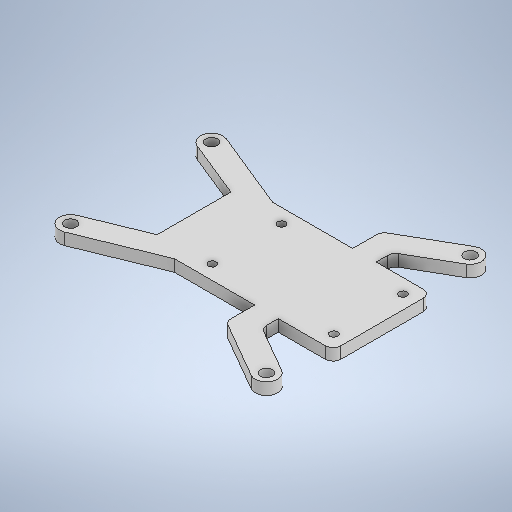
# Autodesk Inventor part: base_c
Saved by Autodesk Inventor 2025.2 (Build 292293000, 293)
## iProperties
Created: 2025-03-26
Part Number: base_c
Material: Generic
Document SubType Name: Modeling
Designer: cdavi
Density: 1 g/cm^3
Appearance: Default
Mass: 4.94389 g
Surface Area: 44.1455 cm^2
Volume: 4.94389 cm^3
Author: cdavi
Autodesk Inventor part; units mm, degrees
ref_plane "YZ Plane" through (0, 0, 0) normal (1, 0, 0) x (0, 1, 0)
ref_plane "XZ Plane" through (0, 0, 0) normal (0, 1, 0) x (-1, 0, 0)
ref_plane "XY Plane" through (0, 0, 0) normal (0, 0, 1) x (1, 0, 0)
sketch "Sketch1" plane through (0, 0, 0) normal (0, 1, 0) x (-1, 0, 0)
  line L0 (-29, 26) -> (29, 26)
  line L1 (29, 26) -> (29, -26)
  line L2 (29, -26) -> (-29, -26)
  line L3 (-29, -26) -> (-29, 26)
  line L4 (-29, 26) -> (29, -26) construction
  line L5 (29, 26) -> (-29, -26) construction
  line L6 (-32.5, 29.5) -> (32.5, 29.5)
  line L7 (32.5, -29.5) -> (-32.5, -29.5)
  line L8 (-32.5, -29.5) -> (-32.5, 29.5)
  line L9 (-32.5, 29.5) -> (32.5, -29.5) construction
  line L10 (32.5, 29.5) -> (-32.5, -29.5) construction
  circle A0 centre (-29, 26) radius 1.5
  circle A1 centre (-29, -26) radius 1.5
  line L11 (32.5, 29.5) -> (32.5, 5.9791)
  line L12 (32.5, -5.9791) -> (32.5, -29.5)
  line L13 (29, 0) -> (29, -18)
  circle A2 centre (29, -18) radius 1.5
  arc A3 (32.5, 5.9791) -> (32.5, -5.9791) centre (33, 0) ccw
  line L14 (32.5, -5.9791) -> (32.5, 5.9791)
  line L15 (33, 0) -> (-32.5, 0)
  line L16 (29, 0) -> (29, 18)
  circle A4 centre (29, 18) radius 1.5
  point P0 (0, 0)
  dimension "d1" = 58
  dimension "d3" = 3.5
  dimension "d7" = 3
  dimension "d8" = 3
  dimension "d31" = 52
  dimension "d32" = 3.5
  dimension "d33" = 18
  dimension "d34" = 3
  constraints: 34 end point, 6 midpoint, 5 centre point, 5 parallel, 4 coincident, 3 perpendicular, 2 horizontal, 2 point on circle, 2 symmetric about line, 1 point on line, 1 vertical, 2 other
  measures "d1" distance of L0.start L0.end
  measures "d3" distance between parallel lines of L7 L2
  measures "d7" diameter of A0
  measures "d8" diameter of A1
  measures "d31" distance of L0.end L1.end
  measures "d32" distance between parallel lines of L1 L11
  measures "d33" distance of L13.start L13.end
  measures "d34" diameter of A2
ref_plane "Work Plane1" through (0, 3, 0) normal (0, 1, 0) x (1, 0, 0)
extrude "Extrusion4" add sketch "Sketch1" along normal blind 3 contours A0 L3 L15 L8 L6 L11 A3 L1 A4 L0 | L0 L1 A4 A3 L15 L3 A0 | L15 A3 L1 A2 L2 A1 L3 | L3 A1 L2 L1 A2 A3 L12 L7 L8 L15
sketch "Sketch3" plane through (0, 3, 0) normal (0, 1, 0) x (1, 0, 0)
  circle A0 centre (-29, 18) radius 1.5 projected
  circle A1 centre (-29, 18) radius 2.85
  circle A2 centre (29, 26) radius 1.5 projected
  line L0 (32.5, -29.5) -> (32.5, 29.5) projected
  line L1 (32.5, 0) -> (-15.5, 0)
  line L2 (-15.5, 0) -> (-15.5, 12.5)
  line L3 (-15.5, 12.5) -> (32.5, 12.5)
  line L4 (32.5, 12.5) -> (32.5, 0)
  line L5 (32.5, 0) -> (32.5, 12.5)
  line L6 (32.5, 0) -> (29, 0)
  line L7 (29, 0) -> (29, 8.825)
  line L8 (29, 8.825) -> (-1.99, 8.825)
  line L9 (-1.99, 8.825) -> (-1.99, 0)
  circle A3 centre (-1.99, 8.825) radius 1
  circle A4 centre (29, 8.825) radius 1
  line L10 (-15.5, 0) -> (-15.5, -12.5)
  line L11 (-15.5, -12.5) -> (32.5, -12.5)
  line L12 (32.5, -12.5) -> (32.5, 0)
  line L13 (29, 0) -> (29, -8.825)
  line L14 (29, -8.825) -> (-1.99, -8.825)
  line L15 (-1.99, -8.825) -> (-1.99, 0)
  circle A5 centre (-1.99, -8.825) radius 1
  circle A6 centre (29, -8.825) radius 1
  line L16 (32.5, 26) -> (32.5, 12.5)
  line L17 (-29, 18) -> (-15.5, 12.5)
  line L18 (-30.0753, 15.3606) -> (-15.5, 9.4226)
  line L19 (-27.9247, 20.6394) -> (-13.3494, 14.7013)
  line L20 (32.5, 26) -> (32.5, 12.5)
  line L21 (-13.3494, 14.7013) -> (-7.9463, 12.5)
  circle A7 centre (-29, -18) radius 2.85
  line L22 (-29, -18) -> (-15.5, -12.5)
  line L23 (-30.0753, -15.3606) -> (-15.5, -9.4226)
  line L24 (-27.9247, -20.6394) -> (-13.3494, -14.7013)
  line L25 (-13.3494, -14.7013) -> (-7.9463, -12.5)
  circle A8 centre (29, 26) radius 2.85
  line L26 (32.5, 12.5) -> (15.5, 12.5)
  line L27 (15.5, 12.5) -> (15.5, 18.2058)
  line L28 (15.5, 18.2058) -> (29, 26)
  line L29 (29, 26) -> (27.575, 28.4682)
  line L30 (29, 26) -> (30.425, 23.5318)
  line L31 (27.575, 28.4682) -> (12.5, 19.7646)
  line L32 (12.5, 19.7646) -> (12.5, 12.5)
  line L33 (30.425, 23.5318) -> (18.5, 16.6469)
  line L34 (18.5, 16.6469) -> (18.5, 12.5)
  circle A9 centre (29, -26) radius 2.85
  line L35 (15.5, -12.5) -> (15.5, -18.2058)
  line L36 (15.5, -18.2058) -> (29, -26)
  line L37 (29, -26) -> (27.575, -28.4682)
  line L38 (29, -26) -> (30.425, -23.5318)
  line L39 (27.575, -28.4682) -> (12.5, -19.7646)
  line L40 (12.5, -19.7646) -> (12.5, -12.5)
  line L41 (30.425, -23.5318) -> (18.5, -16.6469)
  line L42 (18.5, -16.6469) -> (18.5, -12.5)
  point P0 (0, 0)
  point P1 (-27.9247, 20.6394)
  point P2 (-27.9247, -20.6394)
  point P3 (-7.9463, -12.5)
  point P4 (15.35, 14.8283)
  point P5 (15.35, -14.8283)
  point P6 (18.5, 12.5)
  point P7 (30.425, 23.5318)
  point P8 (12.5, -12.5)
  point P9 (30.425, -23.5318)
  point P10 (18.5, -12.5)
  point P11 (32.5, -12.5)
  dimension "d37" = 5.7
  dimension "d48" = 5.7
  dimension "d38" = 48
  dimension "d39" = 12.5
  dimension "d40" = 3.5
  dimension "d41" = 8.825
  dimension "d42" = 30.99
  dimension "d43" = 2
  dimension "d44" = 2
  dimension "d49" = 17
  dimension "d50" = 120
  dimension "d51" = 3
  dimension "d52" = 120
  constraints: 84 end point, 28 symmetric about line, 8 point on line, 7 coincident, 5 perpendicular, 4 centre point, 4 horizontal, 3 collinear, 3 parallel, 2 vertical, 1 midpoint, 16 other
  measures "d38" distance of L1.start L1.end
  measures "d39" distance of L1.end L2.end
  measures "d40" distance of L1.start L6.end
  measures "d41" distance of L6.end L7.end
  measures "d42" distance of L7.end L8.end
  measures "d43" diameter of A3
  measures "d44" diameter of A4
  measures "d49" distance of L3.end L26.end
  measures "d50" angle of L27 L28
  measures "d51" distance between parallel lines of L27 L32
  measures "d52" angle of L33 L34
extrude "Extrusion6" cut sketch "Sketch3" against normal blind 10 contours A1 | A1 L19 L21 L3 L17 | L17 L2 L18 A1 | L3 L0 L1 L7 A4 L8 A3 L9 L2 | L1 L15 A5 L14 A6 L13 L0 L11 L10 | L32 L31 A8 L28 L27 L3 | L9 A3 L8 A4 L7 L1 | L1 L13 A6 L14 A5 L15 | L10 L22 A7 L23 | L27 L28 A8 L33 L34 L3 | L11 L25 L24 A7 L22 | A7 | L29 A2 L28 A8 | A8 L30 A2 L29 | L28 A2 L30 A8 | L11 L35 L36 A9 L39 L40 | L42 L41 A9 L36 L35 L11 | L37 L38 A9 | A9 L36 L37 | L38 L36 A9 keep common part
fillet "Fillet3" radius 2 6 edges at (32.5, 1.5, 12.5) (32.5, 1.5, -12.5) (12.5, 1.5, 19.7646) (18.5, 1.5, 16.6469) (18.5, 1.5, -16.6469) (12.5, 1.5, -19.7646)
body "Solid2"
